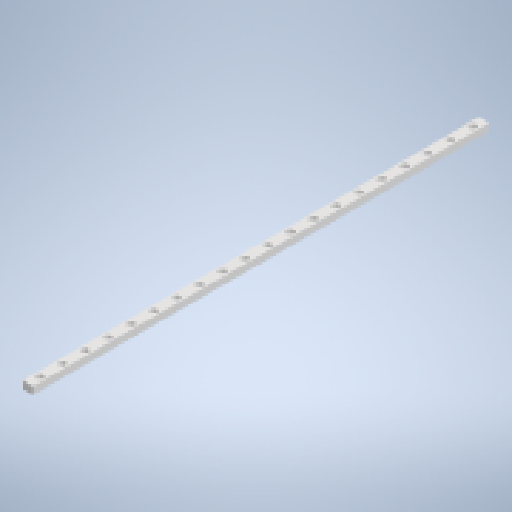
# Autodesk Inventor part: Rail
Saved by Autodesk Inventor 2023 (Build 270158000, 158)
## iProperties
Created: 2022-09-16
Part Number: Rail
Material: Generic
Document SubType Name: Modeling
Designer: deli
Density: 1 g/cm^3
Appearance: Default
Author: deli
Autodesk Inventor part; units mm, degrees
ref_plane "YZ Plane" through (0, 0, 0) normal (1, 0, 0) x (0, 1, 0)
ref_plane "XZ Plane" through (0, 0, 0) normal (0, 1, 0) x (-1, 0, 0)
ref_plane "XY Plane" through (0, 0, 0) normal (0, 0, 1) x (1, 0, 0)
sketch "Sketch1" plane through (0, 0, 0) normal (0, 1, 0) x (-1, 0, 0)
  line L0 (8.568, 23.633) -> (-0.432, 23.633)
  line L1 (-0.432, 23.633) -> (-0.432, -376.367)
  line L2 (-0.432, -376.367) -> (8.568, -376.367)
  line L3 (8.568, -376.367) -> (8.568, 23.633)
  circle A0 centre (4.068, 13.633) radius 1.75
  circle A1 centre (4.068, -6.367) radius 1.75
  circle A2 centre (4.068, -26.367) radius 1.75
  circle A3 centre (4.068, -46.367) radius 1.75
  circle A4 centre (4.068, -66.367) radius 1.75
  circle A5 centre (4.068, -86.367) radius 1.75
  circle A6 centre (4.068, -106.367) radius 1.75
  circle A7 centre (4.068, -126.367) radius 1.75
  circle A8 centre (4.068, -146.367) radius 1.75
  circle A9 centre (4.068, -166.367) radius 1.75
  circle A10 centre (4.068, -186.367) radius 1.75
  circle A11 centre (4.068, -206.367) radius 1.75
  circle A12 centre (4.068, -226.367) radius 1.75
  circle A13 centre (4.068, -246.367) radius 1.75
  circle A14 centre (4.068, -266.367) radius 1.75
  circle A15 centre (4.068, -286.367) radius 1.75
  circle A16 centre (4.068, -306.367) radius 1.75
  circle A17 centre (4.068, -326.367) radius 1.75
  circle A18 centre (4.068, -346.367) radius 1.75
  circle A19 centre (4.068, -366.367) radius 1.75
  point P0 (0, 0)
  dimension "d0" = 9
  dimension "d1" = 400
  dimension "d2" = 3.5
  dimension "d3" = 4.5
  dimension "d7" = 20
  dimension "d12" = 380
  dimension "d13" = 10
  constraints: 20 centre point, 8 end point, 2 parallel, 1 horizontal, 1 perpendicular, 1 vertical, 38 other
  measures "d0" distance of L0.start L0.end
  measures "d1" distance of L2.end L0.start
  measures "d2" diameter of A0
  measures "d3" distance from line of L3 A0.centre
  measures "d7" distance of A0.centre A1.centre
  measures "d12" distance of A19.centre A0.centre
  measures "d13" distance from line of A0.centre L0
extrude "Extrusion1" add sketch "Sketch1" along normal blind 6.5
sketch "Sketch2" plane through (0, 6.5, 0) normal (0, 1, 0) x (1, 0, 0)
  circle A0 centre (-4.068, -13.633) radius 1.75 construction
  circle A1 centre (-4.068, 6.367) radius 1.75 construction
  circle A2 centre (-4.068, -13.633) radius 3
  line L0 (-8.568, 376.367) -> (-8.568, -23.633) construction
  circle A3 centre (-4.068, 6.367) radius 3
  circle A4 centre (-4.068, 26.367) radius 3
  circle A5 centre (-4.068, 46.367) radius 3
  circle A6 centre (-4.068, 66.367) radius 3
  circle A7 centre (-4.068, 86.367) radius 3
  circle A8 centre (-4.068, 106.367) radius 3
  circle A9 centre (-4.068, 126.367) radius 3
  circle A10 centre (-4.068, 146.367) radius 3
  circle A11 centre (-4.068, 166.367) radius 3
  circle A12 centre (-4.068, 186.367) radius 3
  circle A13 centre (-4.068, 206.367) radius 3
  circle A14 centre (-4.068, 226.367) radius 3
  circle A15 centre (-4.068, 246.367) radius 3
  circle A16 centre (-4.068, 266.367) radius 3
  circle A17 centre (-4.068, 286.367) radius 3
  circle A18 centre (-4.068, 306.367) radius 3
  circle A19 centre (-4.068, 326.367) radius 3
  circle A20 centre (-4.068, 346.367) radius 3
  circle A21 centre (-4.068, 366.367) radius 3
  point P0 (0, 0)
  dimension "d16" = 20
  dimension "d17" = 6
  dimension "d20" = 20
  constraints: 20 centre point, 1 coincident, 1 vertical, 38 other
  measures "d16" distance of A1.centre A0.centre
  measures "d17" diameter of A2
  measures "d20" distance of A2.centre A3.centre
extrude "Extrusion2" cut sketch "Sketch2" against normal blind 3.5
equation "\"d3\" = 0.5 * d0"
equation "\"d13\" = -0.5 * d12 + 0.5 * d1"
equation "\"d20\" = d16"
body "Solid1"
